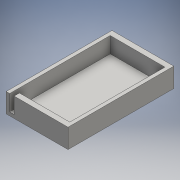
# Autodesk Inventor part: prueba1Bateria
Saved by Autodesk Inventor 2016 (Build 200138000, 138)
## iProperties
Created: 2016-04-24
Part Number: prueba1Bateria
Material: Generic
Document SubType Name: Modeling
Designer: Freddy Chang
Density: 1 g/cm^3
Appearance: Default
Author: Freddy Chang
Autodesk Inventor part; units mm, degrees
ref_plane "YZ Plane" through (0, 0, 0) normal (1, 0, 0) x (0, 1, 0)
ref_plane "XZ Plane" through (0, 0, 0) normal (0, 1, 0) x (-1, 0, 0)
ref_plane "XY Plane" through (0, 0, 0) normal (0, 0, 1) x (1, 0, 0)
sketch "Sketch1" plane through (0, 0, 0) normal (0, 0, 1) x (1, 0, 0)
  line L0 (0, 0) -> (35.08, 0)
  line L1 (35.08, 0) -> (35.08, -60)
  line L2 (35.08, -60) -> (0, -60)
  line L3 (0, -60) -> (0, 0)
  dimension "d0" = 35.08
  dimension "d1" = 60
  constraints: 8 end point, 2 parallel, 1 horizontal, 1 perpendicular
  measures "d0" distance of L1.end L2.end
  measures "d1" distance of L0.end L1.end
extrude "Extrusion1" add sketch "Sketch1" along normal blind 11
sketch "Sketch2" plane through (0, 0, 11) normal (0, 0, 1) x (1, 0, 0)
  line L0 (2, -3) -> (33.08, -3)
  line L1 (33.08, -3) -> (33.08, -57)
  line L2 (33.08, -57) -> (2, -57)
  line L3 (2, -57) -> (2, -3)
  line L4 (0, 0) -> (35.08, 0) projected
  line L5 (0, -60) -> (35.08, -60) projected
  line L6 (35.08, 0) -> (35.08, -60) projected
  line L7 (0, 0) -> (0, -60) projected
  dimension "d8" = 3
  dimension "d9" = 3
  dimension "d10" = 2
  dimension "d11" = 2
  constraints: 8 end point, 2 parallel, 1 horizontal, 1 perpendicular
  measures "d8" distance between parallel lines of L4 L0
  measures "d9" distance between parallel lines of L5 L2
  measures "d10" distance between parallel lines of L6 L1
  measures "d11" distance between parallel lines of L7 L3
extrude "Extrusion2" cut sketch "Sketch2" against normal blind 9 contours L0 L1 L2 L3
sketch "Sketch4" plane through (0, -60, 0) normal (0, -1, 0) x (1, 0, 0)
  line L0 (2, 11) -> (2, 2) projected
  line L1 (2, 11) -> (2, 2)
  line L2 (2, 2) -> (4.5, 2)
  line L3 (2, 2) -> (33.08, 2) projected
  line L4 (4.5, 2) -> (4.5, 11)
  line L5 (2, 11) -> (4.5, 11)
  line L6 (0, 0) -> (0, 11) projected
  dimension "d22" = 9
  dimension "d23" = 4.5
  constraints: 8 end point, 1 collinear, 1 perpendicular, 1 point on line
  measures "d22" distance of L2.end L4.end
  measures "d23" distance between parallel lines of L6 L4
extrude "Extrusion3" cut sketch "Sketch4" against normal blind 3
body "Solid1"
